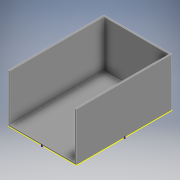
# Autodesk Inventor part: Component box Bottom tall
Saved by Autodesk Inventor 2021 (Build 250183000, 183)
## iProperties
Created: 2023-01-12
Part Number: Component box Bottom tall
Material: Generic
Document SubType Name: Modeling
Designer: boyle
Density: 1 g/cm^3
Appearance: Default
Author: boyle
Autodesk Inventor part; units mm, degrees
ref_plane "YZ Plane" through (0, 0, 0) normal (1, 0, 0) x (0, 1, 0)
ref_plane "XZ Plane" through (0, 0, 0) normal (0, 1, 0) x (-1, 0, 0)
ref_plane "XY Plane" through (0, 0, 0) normal (0, 0, 1) x (1, 0, 0)
sketch "Sketch1" plane through (0, 0, 0) normal (0, 1, 0) x (-1, 0, 0)
  line L0 (0, 0) -> (-177.8, 0)
  line L1 (-177.8, 0) -> (-177.8, 254)
  line L2 (-177.8, 254) -> (0, 254)
  line L3 (0, 254) -> (0, 0)
  dimension "d0" = 177.8
  dimension "d1" = 254
  constraints: 8 end point, 2 parallel, 1 horizontal, 1 perpendicular
  measures "d0" distance of L1.end L2.end
  measures "d1" distance of L0.end L1.end
extrude "Extrusion1" add sketch "Sketch1" along normal blind 127
shell "Shell1" thickness 3.81 removed faces 1 at (118.5333, 127, 169.3333)
sketch "Sketch2" plane through (0, 0, 254) normal (0, 0, 1) x (1, 0, 0)
  line L0 (0, 0) -> (177.8, 0) projected
  line L1 (177.8, 0) -> (177.8, 127) projected
  line L2 (0, 127) -> (177.8, 127) projected
  line L3 (0, 0) -> (0, 127) projected
extrude "Extrusion2" cut sketch "Sketch2" against normal up to surface (3.81 mm away)
sketch "Sketch3" plane through (0, 0, 0) normal (0, -1, 0) x (1, 0, 0)
  line L0 (177.8, 250.19) -> (0, 250.19) projected
  line L1 (0, 0) -> (0, 250.19) projected
  line L2 (177.8, 0) -> (0, 0) projected
  line L3 (177.8, 250.19) -> (177.8, 0) projected
  line L4 (177.8, 250.19) -> (0, 250.19) projected
  line L5 (0, 0) -> (0, 250.19) projected
  line L6 (177.8, 0) -> (0, 0) projected
  line L7 (177.8, 250.19) -> (177.8, 0) projected
  line L8 (177.8, 250.19) -> (177.8, 0) projected
  spline S0 degree 4 poles (88.9, 250.19) (64.6184, 235.605) (118.3851, 244.1086) (81.3712, 187.8473) (79.1664, 164.6282) (100.7722, 157.4816) (94.5532, 141.1288) (75.1172, 136.7588) (92.4319, 127.4973) (95.6269, 113.3719) (72.1361, 104.6051) (96.8499, 82.5804) (92.3371, 68.5262) (76.0031, 58.8905) (95.1922, 46.8111) (88.2393, 30.5759) (70.5928, 15.1042) (112.5447, 15.7388) (88.9, 0) knots 0 0 0 0 0 0.160311 0.22783 0.291752 0.343709 0.393485 0.441731 0.491587 0.546869 0.603873 0.660906 0.71719 0.768135 0.818353 0.868814 1 1 1 1 1
  spline S1 degree 4 poles (0, 125.095) (-6.7527, 130.6116) (46.7852, 140.872) (29.9087, 101.3612) (79.7395, 129.7272) (116.5747, 129.6492) (130.5567, 112.1302) (157.3819, 135.4422) (165.3765, 119.4615) (177.8, 125.095) knots 0 0 0 0 0 0.260408 0.392164 0.513635 0.63886 0.751218 1 1 1 1 1
  point P0 (83.696, 239.0199)
  point P1 (95.7292, 222.4771)
  point P2 (82.8296, 179.2151)
  point P3 (85.8648, 164.5428)
  point P4 (95.9821, 154.1745)
  point P5 (91.1764, 142.7929)
  point P6 (82.3237, 135.7143)
  point P7 (88.9, 127.3714)
  point P8 (91.4293, 116.2479)
  point P9 (82.0708, 103.6056)
  point P10 (91.9352, 81.8518)
  point P11 (88.9, 68.1851)
  point P12 (83.0825, 58.3094)
  point P13 (90.6705, 46.414)
  point P14 (88.9, 35.0509)
  point P15 (83.696, 23.6656)
  point P16 (92.3673, 15.4774)
  point P17 (7.7387, 130.6712)
  point P18 (36.1302, 125.095)
  point P19 (45.4777, 117.014)
  point P20 (78.8552, 125.095)
  point P21 (117.0831, 125.095)
  point P22 (130.5534, 121.195)
  point P23 (147.0022, 125.095)
  point P24 (161.5605, 125.095)
  point P25 (177.8, 125.095)
  point P26 (88.946, 127.3179)
  point P27 (88.9, 250.19)
  point P28 (88.9, 0)
  point P29 (0, 127.787)
  constraints: 4 midpoint, 29 other
body "Solid1"
